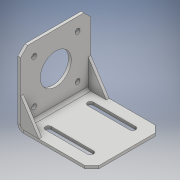
# Autodesk Inventor part: SuporteLMotorNema17
Saved by Autodesk Inventor 2018 (Build 220112000, 112)
## iProperties
Created: 2018-09-20
Part Number: SuporteLMotorNema17
Material: Genérico
Document SubType Name: Chapa de metal
Designer: Georgines
Density: 1 g/cm^3
Sheet Metal Rule: Padrão_mm
Sheet Metal Width: 0,000 mm
Sheet Metal Length: 0,000 mm
Sheet Metal Area: 0,000 mm^2
Appearance: Padrão
Author: Georgines
Autodesk Inventor part; units mm, degrees
ref_plane "YZ Plane" through (0, 0, 0) normal (1, 0, 0) x (0, 1, 0)
ref_plane "XZ Plane" through (0, 0, 0) normal (0, 1, 0) x (-1, 0, 0)
ref_plane "XY Plane" through (0, 0, 0) normal (0, 0, 1) x (1, 0, 0)
sketch "Esboço10" plane through (-2.7381, 25, 4) normal (0, 1, 0) x (1, 0, 0)
  line L0 (47.7381, 2) -> (4, 2)
  line L1 (15, 2) -> (4, 2)
  line L2 (2, 0) -> (2, -18)
  line L3 (2, 0) -> (2, -41.7381)
  line L4 (15, 2) -> (2, -18)
  arc A0 (4, 2) -> (2, 0) centre (4, 0) ccw
  point P0 (2.7381, 4)
  point P1 (2, 2)
  dimension "d59" = 20
  dimension "d60" = 13
  dimension "d61" = 2
  measures "d59" distance of point (2, 2) L2.end
  measures "d60" distance of L1.start point (2, 2)
  measures "d61" radius of A0
sketch "Esboço12" plane through (-2.7381, -25, 4) normal (0, -1, 0) x (1, 0, 0)
  line L0 (2, 18) -> (15, -2)
  line L1 (15, -2) -> (4, -2)
  line L2 (2, 0) -> (2, 41.7381)
  line L3 (2, 0) -> (2, 18)
  line L4 (2, 18) -> (15, -2)
  arc A0 (2, 0) -> (4, -2) centre (4, 0) ccw
  point P0 (2.7381, -4)
  point P1 (2, -2)
  dimension "d64" = 20
  dimension "d65" = 2
  measures "d64" distance of point (2, -2) L3.end
  measures "d65" radius of A0
sketch "Esboço1" plane through (0, 0, 0) normal (0, 0, 1) x (1, 0, 0)
  line L0 (-50, 25) -> (50, 25)
  line L1 (50, 25) -> (50, -25)
  line L2 (50, -25) -> (-50, -25)
  line L3 (-50, -25) -> (-50, 25)
  line L4 (-50, 25) -> (50, -25) construction
  point P0 (0, 0)
  dimension "d0" = 100
  dimension "d1" = 50
  measures "d0" distance of L1.end L2.end
  measures "d1" distance of L0.end L1.end
extrude "Placa1" add sketch "Esboço1" along normal blind 2
chamfer "Chanfro1" distance 5 angle 45 4 edges at (-50, 25, 1) (-50, -25, 1) (50, 25, 1) (50, -25, 1)
sketch "Esboço4" plane through (0, 0, 2) normal (0, 0, 1) x (1, 0, 0)
  line L0 (-45, 25) -> (45, 25) projected
  line L1 (-1, 25) -> (-1, -25)
  line L2 (45, -25) -> (-45, -25) projected
  line L3 (50, 20) -> (50, -20) projected
  point P0 (0, 0)
  dimension "d16" = 51
  constraints: 2 end point, 2 point on line, 1 vertical
  measures "d16" distance between parallel lines of L3 L1
fold "Dobra2" angle 90 bend radius 2 thickness 2 k factor 0.44 line from (-1, 25, 2) to (-1, -25, 2) line at bend centre moving side (-1, 0, 0) folds toward (0, 0, 1)
sketch "Esboço5" plane through (0, 0, 2) normal (0, 0, 1) x (1, 0, 0)
  line L0 (39, 24.4468) -> (39, -25) construction
  line L1 (45, -25) -> (1.2619, -25) construction
  line L2 (50, 20) -> (50, -20) construction
  line L3 (50, 0) -> (1.2619, 0) construction
  line L4 (1.2619, 25) -> (1.2619, -25) construction
  line L5 (50, 15) -> (1.2619, 15) construction
  line L6 (50, -15) -> (1.2619, -15) construction
  line L7 (39, 15) -> (9, 15) construction
  line L8 (39, 17.1) -> (9, 17.1)
  line L9 (9, 12.9) -> (39, 12.9)
  arc A0 (39, 12.9) -> (39, 17.1) centre (39, 15) ccw
  arc A1 (9, 17.1) -> (9, 12.9) centre (9, 15) ccw
  line L10 (39, -15) -> (9, -15) construction
  line L11 (39, -12.9) -> (9, -12.9)
  line L12 (9, -17.1) -> (39, -17.1)
  arc A2 (39, -17.1) -> (39, -12.9) centre (39, -15) ccw
  arc A3 (9, -12.9) -> (9, -17.1) centre (9, -15) ccw
  point P0 (0, 0)
  point P1 (24, 15)
  point P2 (24, -15)
  dimension "d23" = 11
  dimension "d24" = 15
  dimension "d25" = 15
  dimension "d26" = 30
  dimension "d27" = 4.2
  dimension "d28" = 30
  dimension "d29" = 4.2
  constraints: 24 end point, 11 point on line, 8 point on circle, 8 tangent, 4 centre point, 4 midpoint, 2 parallel, 2 perpendicular, 1 vertical
  measures "d23" distance between parallel lines of L2 L0
  measures "d24" distance between parallel lines of L3 L5
  measures "d25" distance between parallel lines of L3 L6
  measures "d26" distance of L7.start L7.end
  measures "d27" diameter of A1
  measures "d28" distance of L10.start L10.end
  measures "d29" diameter of A3
extrude "Recortar1" cut sketch "Esboço5" against normal blind 2
sketch "Esboço6" plane through (-2.7381, -20, 50.7381) normal (-1, 0, 0) x (0, 0, 1)
  line L0 (0, 0) -> (0, 40) projected
  line L1 (0, 20) -> (-49, 20) construction
  line L2 (-24.5, -5) -> (-24.5, 45) construction
  circle A0 centre (-24.5, 20) radius 11.05
  point P0 (-50.7381, 20)
  dimension "d32" = 49
  dimension "d33" = 24.5
  dimension "d34" = 22.1
  constraints: 4 end point, 2 midpoint, 1 centre point, 1 horizontal
  measures "d32" distance of L1.start L1.end
  measures "d33" distance between parallel lines of L2 L0
  measures "d34" diameter of A0
extrude "Recortar2" cut sketch "Esboço6" against normal blind 2
sketch "Esboço7" plane through (-2.7381, -20, 50.7381) normal (-1, 0, 0) x (0, 0, 1)
  line L0 (-46.7381, -5) -> (-5, -5) projected
  line L1 (-24.5608, -5) -> (-24.5608, 43.1749) construction
  line L2 (0, 0) -> (0, 40) construction
  line L3 (0, 20) -> (-49, 20) construction
  circle A0 centre (-9.0608, 35.5) radius 1 construction
  circle A1 centre (-9.0608, 4.5) radius 1 construction
  circle A2 centre (-40.0608, 4.5) radius 1 construction
  circle A3 centre (-40.0608, 35.5) radius 1 construction
  point P0 (-50.7381, 20)
  dimension "d23" = 11
  dimension "d37" = 49
  dimension "d38" = 2
  dimension "d39" = 2
  dimension "d40" = 2
  dimension "d41" = 2
  dimension "d42" = 15.5
  dimension "d43" = 15.5
  dimension "d44" = 15.5
  dimension "d45" = 15.5
  dimension "d46" = 15.5
  dimension "d47" = 15.5
  dimension "d48" = 15.5
  dimension "d49" = 15.5
  constraints: 4 centre point, 4 end point, 1 horizontal, 1 midpoint, 1 perpendicular, 1 point on line
  measures "d37" distance of L3.start L3.end
  measures "d38" diameter of A0
  measures "d39" diameter of A1
  measures "d40" diameter of A2
  measures "d41" diameter of A3
  measures "d42" distance from line of A0.centre L3
  measures "d43" distance from line of L1 A0.centre
  measures "d44" distance from line of L3 A1.centre
  measures "d45" distance from line of L1 A1.centre
  measures "d46" distance from line of L1 A2.centre
  measures "d47" distance from line of L1 A3.centre
  measures "d48" distance from line of L3 A3.centre
  measures "d49" distance from line of L3 A2.centre
hole "Furo1" at (-2.7381, 15.5, 41.6773) at (-2.7381, 15.5, 10.6773) at (-2.7381, -15.5, 41.6773) at (-2.7381, -15.5, 10.6773) direction (1, 0, 0) diameter 3.5 end through all
extrude "Placa2" add sketch "Esboço10" against normal blind 2 separate body
extrude "Placa3" add sketch "Esboço12" against normal blind 2 separate body
equation "\"d2\" = Espessura"
equation "\"d17\" = Largura_alívio_de_vergadura"
equation "\"d18\" = Profundidade_alívio_de_vergadura"
equation "\"d19\" = Remanescente_mínimo"
equation "\"d20\" = Raiodetransição"
equation "\"d25\" = d24"
equation "\"d30\" = Espessura"
equation "\"d35\" = Espessura"
equation "\"d44\" = d42"
equation "\"d45\" = d42"
equation "\"d46\" = d43"
equation "\"d47\" = d43"
equation "\"d48\" = d42"
equation "\"d49\" = d42"
equation "\"d55\" = Espessura"
equation "\"d62\" = Espessura"
equation "\"d66\" = Espessura"
equation "\"Raio_vergadura\" = Espessura"
equation "\"Largura_alívio_de_vergadura\" = Espessura"
equation "\"Profundidade_alívio_de_vergadura\" = 0.5 * Espessura"
equation "\"Tamanho_alívio_de_dobra\" = 4 * Espessura"
equation "\"Remanescente_mínimo\" = 2 * Espessura"
equation "\"Raiodetransição\" = Raio_vergadura"
equation "\"Tamanho_de_raio_de_Jacobi\" = Raio_vergadura"
equation "\"TamanhoFolga\" = Espessura"
equation "\"Espessura\" = 2"
